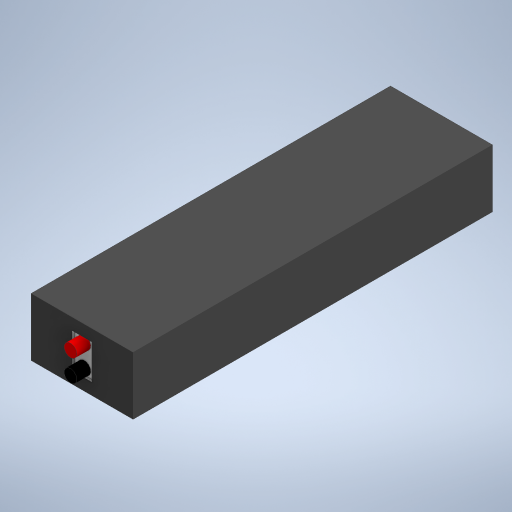
# Autodesk Inventor part: li_pol_3S_5000mAh
Saved by Autodesk Inventor 2023 (Build 270158000, 158)
## iProperties
Created: 2024-07-26
Part Number: li_pol_3S_5000mAh
Material: Ogólny
Document SubType Name: Modeling
Designer: kamil
Density: 1 g/cm^3
Appearance: Domyślna
Author: kamil
Autodesk Inventor part; units mm, degrees
ref_plane "YZ Plane" through (0, 0, 0) normal (1, 0, 0) x (0, 1, 0)
ref_plane "XZ Plane" through (0, 0, 0) normal (0, 1, 0) x (-1, 0, 0)
ref_plane "XY Plane" through (0, 0, 0) normal (0, 0, 1) x (1, 0, 0)
sketch "Szkic1" plane through (0, 0, 0) normal (0, 1, 0) x (-1, 0, 0)
  line L0 (0, 0) -> (44, 0)
  line L1 (44, 0) -> (44, -155)
  line L2 (44, -155) -> (0, -155)
  line L3 (0, -155) -> (0, 0)
  dimension "d0" = 44
  dimension "d1" = 155
  constraints: 8 end point, 2 parallel, 1 horizontal, 1 perpendicular
  measures "d0" distance of L1.end L2.end
  measures "d1" distance of L0.end L1.end
extrude "Wyciągnięcie proste1" add sketch "Szkic1" along normal blind 25
sketch "Szkic2" plane through (-44, 0, 0) normal (0, 0, 1) x (1, 0, 0)
  line L0 (0, 0) -> (44, 0) projected
  line L1 (44, 0) -> (44, 25) projected
  line L2 (0, 25) -> (44, 25) projected
  line L3 (0, 0) -> (0, 25) projected
  line L4 (17.75, 20) -> (26.25, 20)
  line L5 (26.25, 20) -> (26.25, 5)
  line L6 (26.25, 5) -> (17.75, 5)
  line L7 (17.75, 5) -> (17.75, 20)
  circle A0 centre (22, 17.25) radius 2.75
  circle A1 centre (22, 7.75) radius 2.75
  point P0 (26.25, 12.5)
  point P1 (44, 12.5)
  point P2 (22, 20)
  point P3 (22, 25)
  point P4 (22, 5)
  point P5 (22, 20)
  point P6 (22, 5)
  dimension "d4" = 8.5
  dimension "d5" = 15
  dimension "d6" = 5.5
  dimension "d7" = 5.5
  constraints: 8 end point, 5 midpoint, 3 vertical alignment, 2 centre point, 2 parallel, 2 tangent, 1 horizontal, 1 horizontal alignment, 1 perpendicular
  measures "d4" distance of L5.end L6.end
  measures "d5" distance of L4.end L5.end
  measures "d6" diameter of A0
  measures "d7" diameter of A1
extrude "Wyciągnięcie proste2" cut sketch "Szkic2" against normal blind 1 contours L4 L5 L6 L7
extrude "Wyciągnięcie proste3" add sketch "Szkic2" along normal blind 5 contours A1 | A0
